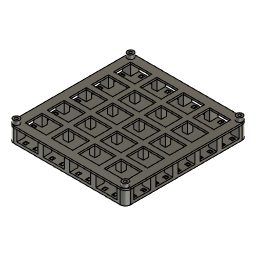
board_holder_outer_ziptie_split_top (Autodesk Fusion 360 design; units mm, degrees)
Autodesk Fusion 360 part; units mm, degrees
note: some values were not read from the file. Chosen so that the rebuilt part matches the saved one: which face or edge a step refers to.
sketch "Sketch1" plane through (0, 0, 0) normal (0, 0, 1) x (1, 0, 0)
  line L0 (-62, -65) -> (62, -65) construction
  line L1 (62, -65) -> (62, 65) construction
  line L2 (62, 65) -> (-62, 65) construction
  line L3 (-62, 65) -> (-62, -65) construction
  line L4 (-62, -65) -> (62, 65) construction
  line L5 (62, -65) -> (-62, 65) construction
  circle A0 centre (-62, 65) radius 1.6
  circle A1 centre (62, 65) radius 1.6
  circle A2 centre (-62, -65) radius 1.6
  circle A3 centre (62, -65) radius 1.6
  line L6 (-66.5, 69.5) -> (66.5, 69.5)
  line L7 (66.5, 69.5) -> (66.5, -69.5)
  line L8 (66.5, -69.5) -> (-66.5, -69.5)
  line L9 (-66.5, -69.5) -> (-66.5, 69.5)
  line L10 (-66.5, 69.5) -> (66.5, -69.5) construction
  line L11 (66.5, 69.5) -> (-66.5, -69.5) construction
  circle A4 centre (-62, 65) radius 3.6
  circle A5 centre (62, 65) radius 3.6
  circle A6 centre (-62, -65) radius 3.6
  circle A7 centre (62, -65) radius 3.6
  dimension "d1" = 124
  dimension "d2" = 130
  dimension "d3" = 3.2
  dimension "d6" = 124
  dimension "d8" = 133
  dimension "d9" = 7.2
  dimension "d12" = 124
  dimension "d102" = 139
  constraint perpendicular L0 L1
  constraint parallel L0 L2
  constraint parallel L1 L3
  constraint horizontal L0
  constraint coincident L4 origin
  constraint coincident L5 origin
  constraint coincident L2.end L3.start
  constraint perpendicular L6 L7
  constraint parallel L6 L8
  constraint parallel L7 L9
  constraint horizontal L6
  constraint coincident L10 origin
  constraint coincident L11 origin
  constraint concentric A0 A4
  measures "d1" distance of L1.end L2.end
  measures "d2" distance of L0.end L1.end
  measures "d3" diameter of A0
  measures "d8" distance of L7.end L8.end
  measures "d9" diameter of A4
  measures "d102" distance of L6.start L8.end L0.start
extrude "Extrude1" add sketch "Sketch1" along normal blind 18.5 contours A4 | A5 | A6 | A7 makes body 1 at (-58.4179, 64.6416, 6.1667) makes body 2 at (65.5821, 64.6416, 6.1667) makes body 3 at (-58.4179, -65.3584, 6.1667) makes body 4 at (65.5821, -65.3584, 6.1667)
extrude "Extrude2" add sketch "Sketch1" against normal blind 3.5 contours L6 L7 L8 L9 | A4 | A5 | A6 | A7 bodies 1 2 3 4
extrude "Extrude3" add sketch "Sketch1" along normal blind 14 contours L6 L7 L8 L9 bodies 1
sketch "Sketch2" plane through (0, -69.5, 0) normal (0, -1, 0) x (1, 0, 0)
  line L0 (66.5, -3.5) -> (66.5, 14)
  line L1 (-66.5, 14) -> (-57, 14)
  line L2 (-57, 14) -> (-57, -3.5)
  line L3 (-57, -3.5) -> (-66.5, -3.5)
  line L4 (-66.5, -3.5) -> (-66.5, 14)
  line L5 (-57, 14) -> (-33, 14)
  line L6 (-33, 14) -> (-33, -3.5)
  line L7 (-33, -3.5) -> (-57, -3.5)
  line L8 (-57, -3.5) -> (-57, 14)
  line L9 (-66.5, 14) -> (-66.5, 12)
  line L10 (-66.5, -3.5) -> (-66.5, 0)
  line L11 (-66.5, 12) -> (66.5, 12)
  line L12 (-66.5, 0) -> (66.5, 0)
  point P0 (-66.5, 14)
  dimension "d64" = 17.5
  dimension "d65" = 9.5
  dimension "d66" = 17.5
  dimension "d67" = 24
  dimension "d68" = 2
  dimension "d69" = 3.5
  constraint horizontal L1
  constraint vertical L2
  constraint horizontal L3
  constraint vertical L4
  constraint horizontal L5
  constraint vertical L6
  constraint horizontal L7
  constraint vertical L8
  constraint perpendicular L1 L9
  constraint perpendicular L3 L10
  constraint coincident L0 L11.end
  constraint perpendicular L0 L11
  constraint coincident L0 L12.end
  constraint perpendicular L0 L12
  constraint coincident P0 L1.start
  measures "d64" distance of P0 L3.end
  measures "d65" distance of P0 L1.end
  measures "d66" distance of L1.end L2.end
  measures "d67" distance of L1.end L5.end
  measures "d68" distance of P0 L9.end
  measures "d69" distance of L3.end L10.end
sketch "Sketch3" plane through (66.5, 0, 0) normal (1, 0, 0) x (0, 1, 0)
  line L0 (-69.5, 14) -> (-69.5, -3.5)
  line L1 (-69.5, -3.5) -> (69.5, -3.5)
  line L2 (69.5, -3.5) -> (69.5, 14)
  line L3 (69.5, 14) -> (-69.5, 14)
  line L4 (-69.5, 14) -> (-60, 14)
  line L5 (-60, 14) -> (-60, -3.5)
  line L6 (-60, -3.5) -> (-69.5, -3.5)
  line L7 (-69.5, -3.5) -> (-69.5, 14)
  line L8 (-60, 14) -> (-40.8, 14)
  line L9 (-40.8, 14) -> (-40.8, -3.5)
  line L10 (-40.8, -3.5) -> (-60, -3.5)
  line L11 (-60, -3.5) -> (-60, 14)
  line L12 (-69.5, 14) -> (-69.5, 12)
  line L13 (-69.5, -3.5) -> (-69.5, 0)
  line L14 (-69.5, 12) -> (69.5, 12)
  line L15 (-69.5, 0) -> (69.5, 0)
  dimension "d85" = 9.5
  dimension "d86" = 17.5
  dimension "d87" = 19.2
  dimension "d88" = 17.5
  dimension "d89" = 2
  dimension "d90" = 3.5
  constraint horizontal L4
  constraint vertical L5
  constraint horizontal L6
  constraint vertical L7
  constraint coincident L0.start L3.end
  constraint horizontal L8
  constraint vertical L9
  constraint horizontal L10
  constraint vertical L11
  constraint perpendicular L3 L12
  constraint coincident L0.end L1.start
  constraint perpendicular L6 L13
  constraint coincident L2 L14.end
  constraint perpendicular L2 L14
  constraint coincident L2 L15.end
  constraint perpendicular L2 L15
  measures "d85" distance of L0.start L4.end
  measures "d86" distance of L0.start L0.end
  measures "d87" distance of L4.end L8.end
  measures "d88" distance of L4.end L5.end
  measures "d89" distance of L0.start L12.end
  measures "d90" distance of L0.end L13.end
sketch "Sketch4" plane through (0, 0, -3.5) normal (0, 0, -1) x (1, 0, 0)
  circle A0 centre (-62, 65) radius 1.6
  circle A1 centre (62, 65) radius 1.6
  line L0 (66.5, 69.5) -> (-66.5, 69.5)
  line L1 (-66.5, 69.5) -> (-66.5, -69.5)
  line L2 (-66.5, -69.5) -> (66.5, -69.5)
  line L3 (66.5, -69.5) -> (66.5, 69.5)
  line L4 (62, 65) -> (35, 65)
  line L5 (35, 65) -> (35, 38)
  line L6 (35, 38) -> (62, 38)
  line L7 (62, 38) -> (62, 65)
  circle A2 centre (35, 38) radius 6.5
  circle A3 centre (-62, -65) radius 1.6
  circle A4 centre (62, -65) radius 1.6
  dimension "d43" = 27
  dimension "d44" = 27
  dimension "d45" = 13
  constraint horizontal L4
  constraint vertical L5
  constraint horizontal L6
  constraint vertical L7
  constraint coincident A1.centre L4.start
  constraint coincident L5.end L6.start
  measures "d43" distance of A1.centre L4.end
  measures "d44" distance of A1.centre L6.end
  measures "d45" diameter of A2
extrude "Extrude10" cut sketch "Sketch3" against normal blind 133 contours L5 L9 L11 L14 L15 bodies 1
pattern_linear "R-Pattern2" count 5 spacing 25.2 along (0, 1, 0) of "Extrude10"
extrude "Extrude9" cut sketch "Sketch2" against normal blind 139 contours L2 L6 L8 L11 L12 bodies 1
pattern_linear "R-Pattern1" count 4 spacing 30 along (1, 0, 0) of "Extrude9"
ref_plane "WorkPlane1" through (0, 0, 14) normal (0, 0, 1) x (1, 0, 0)
sketch "Sketch6" plane through (0, 0, 14) normal (0, 0, 1) x (1, 0, 0)
  line L0 (-66.5, 69.5) -> (66.5, 69.5) construction
  line L1 (66.5, 69.5) -> (66.5, -69.5) construction
  line L2 (66.5, -69.5) -> (-66.5, -69.5) construction
  line L3 (-66.5, -69.5) -> (-66.5, 69.5) construction
  line L4 (-66.5, 69.5) -> (66.5, -69.5) construction
  line L5 (66.5, 69.5) -> (-66.5, -69.5) construction
  line L6 (-66.5, -69.5) -> (-57, -69.5) construction
  line L7 (-57, -69.5) -> (-57, -60) construction
  line L8 (-57, -60) -> (-66.5, -60) construction
  line L9 (-66.5, -60) -> (-66.5, -69.5) construction
  line L10 (-57, -60) -> (-33, -60)
  line L11 (-33, -60) -> (-33, -40.8)
  line L12 (-33, -40.8) -> (-57, -40.8)
  line L13 (-57, -40.8) -> (-57, -60)
  dimension "d106" = 133
  dimension "d107" = 139
  dimension "d108" = 9.5
  dimension "d109" = 9.5
  dimension "d110" = 24
  dimension "d111" = 19.2
  constraint perpendicular L0 L1
  constraint parallel L0 L2
  constraint parallel L1 L3
  constraint horizontal L0
  constraint coincident L4 origin
  constraint coincident L5 origin
  constraint horizontal L6
  constraint vertical L7
  constraint horizontal L8
  constraint vertical L9
  constraint horizontal L10
  constraint vertical L11
  constraint horizontal L12
  constraint vertical L13
  measures "d106" distance of L1.end L2.end
  measures "d107" distance of L0.end L1.end
  measures "d108" distance of L2.end L6.end
  measures "d109" distance of L2.end L8.end
  measures "d110" distance of L7.end L10.end
  measures "d111" distance of L7.end L12.end
extrude "Extrude11" cut sketch "Sketch6" against normal blind 2 bodies 1
pattern_linear "R-Pattern3" count 5 spacing 25.2 along (0, 1, 0) count 4 spacing 30 along (1, 0, 0) of "Extrude11"
fillet "Fillet1" radius 6 4 edges at (-66.5, -69.5, 5.25) (66.5, -69.5, 5.25) (66.5, 69.5, 5.25) (-66.5, 69.5, 5.25) on bodies 1
chamfer "Chamfer3" distance 0.4 angle 45 12 edges at (-63.4917, -65.5786, -3.5) (60.5083, -65.5786, -3.5) (60.5083, 64.4214, -3.5) (-63.4917, 64.4214, -3.5) (0, 69.5, -3.5) (-64.7426, 67.7426, -3.5) (-66.5, 0, -3.5) (-64.7426, -67.7426, -3.5) (0, -69.5, -3.5) (64.7426, -67.7426, -3.5) (66.5, 0, -3.5) (64.7426, 67.7426, -3.5) on bodies 1
ref_plane "WorkPlane2" through (0, -65.5, 0) normal (0, 1, 0) x (0, 0, 1)
sketch "Sketch7" plane through (0, -65.5, 0) normal (0, 1, 0) x (1, 0, 0)
  line L0 (0, 0) -> (-66.5, 0) construction
  line L1 (-66.5, 0) -> (-57, 0) construction
  line L2 (-57, 0) -> (-45, 0) construction
  line L3 (-45, 0) -> (-45, 3.5) construction
  line L4 (-45, 0) -> (-27.625, 0) construction
  line L5 (-45, 0) -> (-49, 0) construction
  line L6 (-45, 3.5) -> (-57, 3.5) construction
  line L7 (-49, 0) -> (-49, 1)
  line L8 (-49, 0) -> (-51.5, 0)
  line L9 (-51.5, 0) -> (-51.5, 1)
  arc A0 (-49, 3.5) -> (-51.5, 1) centre (-49, 1) ccw
  line L10 (-49, 1) -> (-45, 1)
  line L11 (-49, 3.5) -> (-45, 3.5)
  line L12 (-45, 3.5) -> (-45, 1)
  arc A1 (-38.5, 1) -> (-41, 3.5) centre (-41, 1) ccw
  line L13 (-41, 0) -> (-38.5, 0)
  line L14 (-38.5, 0) -> (-38.5, 1)
  line L15 (-41, 0) -> (-41, 1)
  line L16 (-41, 1) -> (-45, 1)
  line L17 (-45, 3.5) -> (-33, 3.5) construction
  line L18 (-41, 3.5) -> (-45, 3.5)
  dimension "d121" = 66.5
  dimension "d122" = 9.5
  dimension "d123" = 12
  dimension "d124" = 3.5
  dimension "d126" = 4
  dimension "d127" = 12
  dimension "d128" = 1
  dimension "d129" = 2.5
  dimension "d130" = 1
  constraint coincident L0.start origin
  constraint horizontal L0
  constraint parallel L0 L1
  constraint parallel L0 L2
  constraint perpendicular L2 L3
  constraint perpendicular L3 L4
  constraint perpendicular L3 L5
  constraint perpendicular L3 L6
  constraint perpendicular L5 L7
  constraint perpendicular L7 L8
  constraint perpendicular L0 L9
  constraint coincident L6 A0.start
  constraint coincident L7.end A0.centre
  constraint coincident L3 L10.end
  constraint perpendicular L3 L10
  constraint symmetric L3.end L12 L6.start
  constraint symmetric L5.end L12 L13.start
  constraint symmetric L6.end L12 L17.end
  constraint symmetric L7.end L12 A1.centre
  constraint symmetric L8.end L12 L13.end
  constraint symmetric L9.end L12 A1.start
  constraint symmetric A0.start L12 A1.end
  constraint symmetric A0 L12 A1
  constraint symmetric L10.end L12 L16.end
  measures "d121" distance of L0.start L0.end
  measures "d122" distance of L0.end L1.end
  measures "d123" distance of L1.end L2.end
  measures "d124" distance of L2.end L3.end
  measures "d126" distance of L2.end L5.end
  measures "d127" distance of L3.end L6.end
  measures "d128" distance of L5.end L7.end
  measures "d129" distance of L5.end L8.end
  measures "d130" distance of L8.end L9.end
extrude "Extrude12" cut sketch "Sketch7" along normal blind 2 bodies 1
extrude "Extrude13" cut sketch "Sketch7" against normal blind 2 bodies 1
chamfer "Chamfer4" distance 1 distance2 1 2 edges at (-51.5, -65.5, 0) (-38.5, -65.5, 0) measured on face at (-43.6667, -48.3667, 0) measured on face at (-43.6667, -48.3667, 0) on bodies 1
fillet "Fillet2" radius 3 2 edges at (-51.5, -65.5, -0.9998) (-38.5, -65.5, -0.9998) on bodies 1
pattern_linear "R-Pattern4" count 4 spacing 30 along (1, 0, 0) count 2 spacing 131.5 along (0, 1, 0) of "Extrude12", "Extrude13", "Chamfer4", "Fillet2"
ref_plane "WorkPlane3" through (62.5, 0, 0) normal (1, 0, 0) x (0, 1, 0)
sketch "Sketch8" plane through (62.5, 0, 0) normal (1, 0, 0) x (0, 1, 0)
  line L0 (0, 0) -> (-69.5, 0) construction
  line L1 (-69.5, 0) -> (-60, 0) construction
  line L2 (-60, 0) -> (-50.4, 0) construction
  line L3 (-50.4, 0) -> (-50.4, -1)
  line L4 (-50.4, 0) -> (-54.4, 0) construction
  line L5 (-54.4, 0) -> (-56.9, 0)
  line L6 (-54.4, 0) -> (-54.4, -1)
  line L7 (-56.9, 0) -> (-56.9, -1)
  arc A0 (-56.9, -1) -> (-54.4, -3.5) centre (-54.4, -1) ccw
  line L8 (-54.4, -1) -> (-56.9, -1) construction
  line L9 (-54.4, -1) -> (-54.4, -3.5) construction
  line L10 (-54.4, -1) -> (-50.4, -1)
  line L11 (-50.4, 0) -> (-50.4, -3.5) construction
  line L12 (-50.4, -3.5) -> (-54.4, -3.5)
  line L13 (-50.4, -3.5) -> (-46.4, -3.5)
  arc A1 (-46.4, -3.5) -> (-43.9, -1) centre (-46.4, -1) ccw
  line L14 (-43.9, 0) -> (-43.9, -1)
  line L15 (-46.4, 0) -> (-43.9, 0)
  line L16 (-46.4, 0) -> (-46.4, -1)
  line L17 (-46.4, -1) -> (-50.4, -1)
  dimension "d143" = 69.5
  dimension "d144" = 9.5
  dimension "d145" = 9.6
  dimension "d146" = 1
  dimension "d147" = 4
  dimension "d148" = 2.5
  dimension "d149" = 1
  dimension "d150" = 1
  dimension "d151" = 90
  dimension "d152" = 3.5
  constraint coincident L0.start origin
  constraint horizontal L0
  constraint parallel L0 L1
  constraint parallel L0 L2
  constraint perpendicular L2 L3
  constraint perpendicular L3 L4
  constraint parallel L2 L5
  constraint perpendicular L0 L6
  constraint perpendicular L2 L7
  constraint coincident L6.end A0.centre
  constraint perpendicular L2 L11
  constraint symmetric L3.end L11 L10.end
  constraint symmetric L4.end L11 L15.start
  constraint symmetric L5.end L11 L14.start
  constraint symmetric L6.end L11 A1.centre
  constraint symmetric L7.end L11 A1.end
  constraint symmetric A0.end L11 L13.end
  constraint symmetric A0 L11 A1
  constraint symmetric L12.start L11 L13.start
  measures "d143" distance of L0.start L0.end
  measures "d144" distance of L0.end L1.end
  measures "d145" distance of L1.end L2.end
  measures "d146" distance of L2.end L3.end
  measures "d147" distance of L2.end L4.end
  measures "d148" distance of L4.end L5.end
  measures "d149" distance of L4.end L6.end
  measures "d150" distance of L5.end L7.end
  measures "d151" angle of L8 L9
  measures "d152" distance of L2.end L11.end
extrude "Extrude14" cut sketch "Sketch8" along normal blind 2 bodies 1
extrude "Extrude15" cut sketch "Sketch8" against normal blind 2 bodies 1
chamfer "Chamfer5" distance 1 distance2 1 2 edges at (62.5, -56.9, 0) (62.5, -43.9, 0) measured on face at (-46.3333, 48.5333, 0) measured on face at (-46.3333, 48.5333, 0) on bodies 1
fillet "Fillet3" radius 3 2 edges at (62.5, -56.9, -0.9998) (62.5, -43.9, -0.9998) on bodies 1
pattern_linear "R-Pattern5" count 5 spacing 25.2 along (0, 1, 0) count 2 spacing 125.5 along (-1, 0, 0) of "Extrude14", "Extrude15", "Chamfer5", "Fillet3"
sketch "Sketch9" plane through (0, 0, -3.5) normal (0, 0, -1) x (1, 0, 0)
  line L0 (-61, 21.2) -> (-65, 21.2)
  line L1 (-65, 21.2) -> (-65, 29.2)
  line L2 (-65, 29.2) -> (-61, 29.2)
  line L3 (-61, 29.2) -> (-61, 21.2)
  line L4 (64.5, -4) -> (60.5, -4)
  line L5 (60.5, -4) -> (60.5, 4)
  line L6 (60.5, 4) -> (64.5, 4)
  line L7 (64.5, 4) -> (64.5, -4)
  line L8 (64.5, 46.4) -> (60.5, 46.4)
  line L9 (60.5, 46.4) -> (60.5, 54.4)
  line L10 (60.5, 54.4) -> (64.5, 54.4)
  line L11 (64.5, 54.4) -> (64.5, 46.4)
  line L12 (-19, -68) -> (-19, -64)
  line L13 (-19, -64) -> (-11, -64)
  line L14 (-11, -64) -> (-11, -68)
  line L15 (-11, -68) -> (-19, -68)
  line L16 (11, 63.5) -> (11, 67.5)
  line L17 (11, 67.5) -> (19, 67.5)
  line L18 (19, 67.5) -> (19, 63.5)
  line L19 (19, 63.5) -> (11, 63.5)
  line L20 (-49, 63.5) -> (-49, 67.5)
  line L21 (-49, 67.5) -> (-41, 67.5)
  line L22 (-41, 67.5) -> (-41, 63.5)
  line L23 (-41, 63.5) -> (-49, 63.5)
  circle A0 centre (-62, -65) radius 2
  circle A1 centre (62, 65) radius 2
  circle A2 centre (-62, 65) radius 2
  circle A3 centre (62, -65) radius 2
  line L24 (-60.5, -69.1) -> (60.5, -69.1)
  arc A4 (60.5, -69.1) -> (66.1, -63.5) centre (60.5, -63.5) ccw
  line L25 (66.1, -63.5) -> (66.1, 63.5)
  arc A5 (66.1, 63.5) -> (60.5, 69.1) centre (60.5, 63.5) ccw
  line L26 (60.5, 69.1) -> (-60.5, 69.1)
  arc A6 (-60.5, 69.1) -> (-66.1, 63.5) centre (-60.5, 63.5) ccw
  line L27 (-66.1, 63.5) -> (-66.1, -63.5)
  arc A7 (-66.1, -63.5) -> (-60.5, -69.1) centre (-60.5, -63.5) ccw
  line L28 (-19, 63.5) -> (-19, 67.5)
  line L29 (-19, 67.5) -> (-11, 67.5)
  line L30 (-11, 67.5) -> (-11, 63.5)
  line L31 (-11, 63.5) -> (-19, 63.5)
  line L32 (-49, -68) -> (-49, -64)
  line L33 (-49, -64) -> (-41, -64)
  line L34 (-41, -64) -> (-41, -68)
  line L35 (-41, -68) -> (-49, -68)
  line L36 (11, -68) -> (11, -64)
  line L37 (11, -64) -> (19, -64)
  line L38 (19, -64) -> (19, -68)
  line L39 (19, -68) -> (11, -68)
  line L40 (64.5, 21.2) -> (60.5, 21.2)
  line L41 (60.5, 21.2) -> (60.5, 29.2)
  line L42 (60.5, 29.2) -> (64.5, 29.2)
  line L43 (64.5, 29.2) -> (64.5, 21.2)
  line L44 (-61, 46.4) -> (-65, 46.4)
  line L45 (-65, 46.4) -> (-65, 54.4)
  line L46 (-65, 54.4) -> (-61, 54.4)
  line L47 (-61, 54.4) -> (-61, 46.4)
  line L48 (-61, -4) -> (-65, -4)
  line L49 (-65, -4) -> (-65, 4)
  line L50 (-65, 4) -> (-61, 4)
  line L51 (-61, 4) -> (-61, -4)
  line L52 (62, 65) -> (34.5, 65) construction
  line L53 (34.5, 65) -> (34.5, 39) construction
  line L54 (34.5, 39) -> (62, 39) construction
  line L55 (62, 39) -> (62, 65) construction
  circle A8 centre (34.5, 39) radius 6.5
  line L56 (41, 63.5) -> (41, 67.5)
  line L57 (41, 67.5) -> (49, 67.5)
  line L58 (49, 67.5) -> (49, 63.5)
  line L59 (49, 63.5) -> (41, 63.5)
  line L60 (41, -68) -> (41, -64)
  line L61 (41, -64) -> (49, -64)
  line L62 (49, -64) -> (49, -68)
  line L63 (49, -68) -> (41, -68)
  line L64 (-61, -29.2) -> (-65, -29.2)
  line L65 (-65, -29.2) -> (-65, -21.2)
  line L66 (-65, -21.2) -> (-61, -21.2)
  line L67 (-61, -21.2) -> (-61, -29.2)
  line L68 (64.5, -54.4) -> (60.5, -54.4)
  line L69 (60.5, -54.4) -> (60.5, -46.4)
  line L70 (60.5, -46.4) -> (64.5, -46.4)
  line L71 (64.5, -46.4) -> (64.5, -54.4)
  line L72 (64.5, -29.2) -> (60.5, -29.2)
  line L73 (60.5, -29.2) -> (60.5, -21.2)
  line L74 (60.5, -21.2) -> (64.5, -21.2)
  line L75 (64.5, -21.2) -> (64.5, -29.2)
  line L76 (-61, -54.4) -> (-65, -54.4)
  line L77 (-65, -54.4) -> (-65, -46.4)
  line L78 (-65, -46.4) -> (-61, -46.4)
  line L79 (-61, -46.4) -> (-61, -54.4)
  dimension "d164" = 26
  dimension "d165" = 27.5
  dimension "d166" = 13
  constraint horizontal L52
  constraint vertical L53
  constraint horizontal L54
  constraint vertical L55
  constraint coincident A1.centre L52.start
  constraint coincident L53.end L54.start
  measures "d164" distance of A1.centre L54.end
  measures "d165" distance of A1.centre L52.end
  measures "d166" diameter of A8
ref_plane "WorkPlane4" through (0, 0, 12) normal (0, 0, 1) x (1, 0, 0)
split "Split1" by plane through (0, 0, 12) normal (0, 0, 1) bodies 1 makes body 5 at (-63.3333, -3.2, 14)
extrude "Extrude17" [suppressed]
extrude "Extrude18" [suppressed]
extrude "Extrude16" [suppressed]
chamfer "Chamfer7" [suppressed]
delete_face "DeleteFace2" [suppressed]
chamfer "Chamfer8" [suppressed]
delete_face "DeleteFace3" [suppressed]
delete_face "DeleteFace4" [suppressed]
equation "d1 = PWidth"
equation "d2 = PLength"
equation "d3 = BoltClearence"
equation "d6 = PWidth"
equation "d7 = -PLength"
equation "d8 = BWidth"
equation "d9 = d3 + 4 mm"
equation "d12 = PWidth"
equation "d13 = -PLength"
equation "d14 = PegH"
equation "d16 = -Bottom"
equation "d18 = InnerHeight + XTop"
equation "BWidth = PWidth + 9 mm"
equation "Ends = 9.5 mm"
equation "InnerWalls = 6 mm"
equation "InnerHeight = 12 mm"
equation "XChamberW = ( ( BWidth - ( Ends * 2 ) - ( InnerWalls * ( XChannels - 1 ) ) ) / XChannels )"
equation "Bottom = 3.5 mm"
equation "XTop = 2 mm"
equation "XChamberH = Bottom + XTop + InnerHeight"
equation "PegH = 22 mm - Bottom"
equation "d64 = XChamberH"
equation "d65 = Ends"
equation "d66 = XChamberH"
equation "d67 = XChamberW"
equation "d68 = XTop"
equation "d69 = Bottom"
equation "XChannels = 4"
equation "d79 = -BLength"
equation "d81 = XChannels"
equation "d83 = -( XChamberW + InnerWalls ) * ( XChannels - 1 )"
equation "d85 = Ends"
equation "d86 = XChamberH"
equation "d87 = YChamberW"
equation "d88 = YChamberH"
equation "d89 = YTop"
equation "d90 = Bottom"
equation "d91 = -BWidth"
equation "d93 = YChannels"
equation "d95 = ( YChamberW + InnerWalls ) * ( YChannels - 1 )"
equation "BLength = PLength + 9 mm"
equation "YChamberW = ( ( BLength - ( Ends * 2 ) - ( InnerWalls * ( YChannels - 1 ) ) ) / YChannels )"
equation "YChamberH = Bottom + XTop + InnerHeight"
equation "YChannels = 5"
equation "d102 = BLength"
equation "PWidth = 124 mm"
equation "PLength = 130 mm"
equation "d105 = InnerHeight + XTop"
equation "d106 = BWidth"
equation "d107 = BLength"
equation "d108 = Ends"
equation "d109 = Ends"
equation "d110 = XChamberW"
equation "d111 = YChamberW"
equation "d112 = -XTop"
equation "d114 = YChannels"
equation "d115 = XChannels"
equation "d116 = ( YChamberW + InnerWalls ) * ( YChannels - 1 )"
equation "d117 = -( XChamberW + InnerWalls ) * ( XChannels - 1 )"
equation "d120 = ( -BLength / 2 ) + ( 4 mm )"
equation "d121 = BWidth / 2"
equation "d122 = Ends"
equation "d123 = XChamberW / 2"
equation "d124 = Bottom"
equation "d127 = XChamberW / 2"
equation "d138 = XChannels"
equation "d140 = ( XChamberW + InnerWalls ) * ( XChannels - 1 )"
equation "d141 = ( YChamberW + InnerWalls ) * ( YChannels ) + ( Ends - 4 mm )"
equation "d142 = ( BWidth / 2 ) - ( 4 mm )"
equation "d143 = BLength / 2"
equation "d144 = Ends"
equation "d145 = YChamberW / 2"
equation "d162 = ( YChamberW + InnerWalls ) * ( YChannels - 1 )"
equation "d163 = ( XChamberW + InnerWalls ) * ( XChannels ) + ( Ends - 4 mm )"
equation "BoltClearence = 3.2 mm"
equation "YTop = XTop"
equation "d178 = InnerHeight"
named bodies: "board_6hc_bottom", "board_6hc_top"
